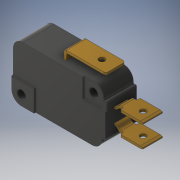
# Autodesk Inventor part: fc17-076
Saved by Autodesk Inventor 2017.1 (Build 211199000, 199)
## iProperties
Category: Electrical
Company: Autodesk Inc.
Created: 2016-12-17
Part Number: fc17-076
Material: Generic
Document SubType Name: Modeling
Designer: Autodesk Inc.
Density: 1 g/cm^3
Appearance: Default
Catalog Web Link: http://www.mouser.com/ds/2/187/honeywell-sensing-micro-switch-V7-basic-product-sh-740331.pdf
Vendor: Honeywell
Author: Autodesk Inc.
Keywords: FIRST Choice
Autodesk Inventor part; units mm, degrees
sketch "Sketch1" plane through (0, 0, 0) normal (0, 1, 0) x (-1, 0, 0)
  line L0 (0, 0) -> (0, -48.4764) construction
  line L1 (0, -48.4764) -> (-27.2974, -48.4764) construction
  line L2 (-27.2974, -48.4764) -> (-27.2974, 0) construction
  line L3 (-27.2974, 0) -> (0, 0) construction
  line L4 (-4.6059, -3.65) -> (-22.1318, -3.65)
  line L5 (-22.1318, -3.65) -> (-22.1318, -32.3372)
  line L6 (-22.1318, -32.3372) -> (-4.6059, -32.3372)
  line L7 (-4.6059, -32.3372) -> (-4.6059, -3.65)
  line L8 (-8.3878, -32.3372) -> (-18.7189, -32.3372)
  line L9 (-18.7189, -32.3372) -> (-18.7189, -33.368)
  line L10 (-18.7189, -33.368) -> (-8.3878, -33.368)
  line L11 (-8.3878, -33.368) -> (-8.3878, -32.3372)
  line L12 (-15.2137, -3.65) -> (-15.2137, -10.9371)
  line L13 (-15.2137, -10.9371) -> (-22.1318, -10.9371)
  line L14 (-10.7861, -32.3372) -> (-10.7861, -26.0648)
  line L15 (-10.7861, -26.0648) -> (-4.6059, -26.0648)
  dimension "d15" = 29.718
  constraints: 24 end point, 5 perpendicular, 5 point on line, 4 parallel, 2 horizontal, 1 vertical, 2 other
  measures "d15" vertical distance of L9.end L4.end
extrude "Extrusion1" add sketch "Sketch1" against normal blind 10.16 contours L7 L15 L14 L6 L5 L13 L12 L4 | L12 L13 L5 L4 | L7 L6 L14 L15
fillet "Fillet1" radius 3.175 4 edges at (4.6059, -5.08, -3.65) (22.1318, -5.08, -3.65) (22.1318, -5.08, -32.3372) (4.6059, -5.08, -32.3372)
extrude "Extrusion2" add sketch "Sketch1" against normal up to surface (10.16 mm away) contours L11 L10 L9 L6
fillet "Fillet2" radius 0.254 4 edges at (8.3878, -5.08, -32.3372) (8.3878, -5.08, -33.368) (18.7189, -5.08, -33.368) (18.7189, -5.08, -32.3372)
sketch "Sketch2" plane through (0, 0, 0) normal (0, 1, 0) x (1, 0, 0)
  arc A0 (7.7809, 32.3372) -> (4.6059, 29.1622) centre (7.7809, 29.1622) ccw projected
  arc A1 (18.9568, 3.65) -> (22.1318, 6.825) centre (18.9568, 6.825) ccw projected
  point P0 (0, 0)
hole "Hole1" at (7.7809, 0, -29.1622) at (18.9568, 0, -6.825) direction (0, -1, 0) diameter 2.794 end through all
sketch "Sketch3" plane through (0, 0, 0) normal (0, 1, 0) x (1, 0, 0)
  arc A0 (7.7809, 32.3372) -> (4.6059, 29.1622) centre (7.7809, 29.1622) ccw projected
  arc A1 (18.9568, 3.65) -> (22.1318, 6.825) centre (18.9568, 6.825) ccw projected
  circle A2 centre (18.9568, 6.825) radius 1.397 projected
  circle A3 centre (7.7809, 29.1622) radius 1.397 projected
  point P0 (0, 0)
sketch "Sketch4" plane through (0, 0, 0) normal (0, 1, 0) x (1, 0, 0)
  line L0 (7.7809, 3.65) -> (18.9568, 3.65) projected
  line L1 (15.242, 3.65) -> (15.242, 3.65)
  line L2 (15.242, 3.65) -> (18.9568, 3.65)
  line L3 (22.1318, 6.825) -> (22.1318, 29.1622) projected
  arc A0 (18.9568, 3.65) -> (22.1318, 6.825) centre (18.9568, 6.825) ccw projected
  line L4 (18.9568, 3.65) -> (15.242, 3.65)
  circle A1 centre (18.9568, 6.825) radius 1.397 projected
  line L5 (15.2137, 3.65) -> (15.2137, 10.9371) projected
  line L6 (15.2137, 10.9371) -> (22.1318, 10.9371) projected
  line L7 (15.2137, 3.65) -> (15.2137, 10.9371)
  line L8 (4.6059, 6.825) -> (4.6059, 29.1622) projected
  line L9 (15.2137, 10.9371) -> (22.1318, 10.9371)
  line L10 (22.1318, 10.9371) -> (22.1318, 6.825)
  line L11 (18.9568, 3.65) -> (15.2137, 3.65)
  point P0 (0, 0)
  constraints: 14 end point, 3 perpendicular, 2 point on circle, 1 collinear, 1 parallel, 1 point on line, 1 tangent, 1 vertical
extrude "Extrusion4" add sketch "Sketch4" along normal blind 0.508
fillet "Fillet3" radius 0.127 4 edges at (15.2137, 0, -7.2936) (15.2137, 0.508, -7.2936) (18.6728, 0, -10.9371) (18.6728, 0.508, -10.9371)
sketch "Sketch6" plane through (0, 0, 0) normal (0, 1, 0) x (1, 0, 0)
  line L0 (4.6059, 26.1612) -> (10.8013, 26.1612)
  line L1 (10.8013, 26.1612) -> (10.8013, 32.3448)
  line L2 (4.6059, 29.1622) -> (4.6059, 26.1612)
  line L3 (10.8013, 32.3448) -> (10.8013, 33.368)
  line L4 (18.4649, 33.368) -> (8.6418, 33.368) projected
  line L5 (10.8013, 33.368) -> (8.6418, 33.368)
  line L6 (4.6059, 29.1622) -> (4.6059, 6.825) projected
  arc A0 (7.7809, 32.3372) -> (4.6059, 29.1622) centre (7.7809, 29.1622) ccw projected
  line L7 (7.7809, 32.3372) -> (8.1338, 32.3372) projected
  line L8 (7.7809, 32.3372) -> (8.1338, 32.3372)
  arc A1 (8.1338, 32.3372) -> (8.3878, 32.5912) centre (8.1338, 32.5912) ccw projected
  line L9 (8.3878, 32.5912) -> (8.3878, 33.114)
  line L10 (8.3878, 33.114) -> (8.3878, 32.5912) projected
  arc A2 (8.1338, 32.3372) -> (8.3878, 32.5912) centre (8.1338, 32.5912) ccw
  arc A3 (8.6418, 33.368) -> (8.3878, 33.114) centre (8.6418, 33.114) ccw projected
  arc A4 (8.6418, 33.368) -> (8.3878, 33.114) centre (8.6418, 33.114) ccw
  point P0 (0, 0)
  constraints: 17 end point, 6 point on circle, 3 collinear, 2 centre point, 2 coincident, 2 concentric, 2 horizontal, 1 parallel, 1 perpendicular, 1 point on line, 1 vertical
extrude "Extrusion5" cut sketch "Sketch6" against normal blind 0.508
fillet "Fillet4" radius 0.127 14 edges at (5.5358, -0.508, -31.4073) (7.9573, -0.508, -32.3372) (8.3134, -0.508, -32.4116) (8.3878, -0.508, -32.8526) (8.4622, -0.508, -33.2936) (9.7215, -0.508, -33.368) (4.6059, -0.508, -27.6617) (10.8013, -0.254, -33.368) (10.8013, 0, -29.7646) (10.8013, -0.508, -29.7646) (10.8013, -0.254, -26.1612) (7.7036, -0.508, -26.1612) (7.7036, 0, -26.1612) (4.6059, -0.254, -26.1612)
ref_plane "Work Plane2" through (9.5334, -10.16, -6.825) normal (-1, 0, 0) x (0, 0, 1)
ref_plane "Work Plane1" through (13.3688, -10.16, -6.825) normal (-1, 0, 0) x (0, 0, 1)
ref_plane "Work Plane3" through (0, -5.08, 0) normal (0, 1, 0) x (1, 0, 0)
sketch "Sketch9" plane through (0, -5.08, 0) normal (0, 1, 0) x (1, 0, 0)
  line L0 (9.5334, -6.6736) -> (9.5334, 40.0416) projected
  circle A0 centre (7.7809, 29.1622) radius 1.397 projected
  line L1 (9.5334, 33.368) -> (9.5334, 42.8385)
  line L2 (10.2954, 33.368) -> (10.2954, 42.8385)
  line L3 (10.6743, 33.368) -> (8.6418, 33.368) projected
  line L4 (10.9283, 33.368) -> (10.6743, 33.368) projected
  line L5 (18.4649, 33.368) -> (10.9283, 33.368) projected
  line L6 (9.7239, 43.6402) -> (10.1049, 43.6402)
  line L7 (9.5334, 42.8385) -> (9.7239, 43.6402)
  line L8 (10.2954, 42.8385) -> (10.1049, 43.6402)
  line L9 (10.2954, 35.0309) -> (11.3926, 34.062)
  line L10 (11.3926, 34.062) -> (11.3926, 33.368)
  line L11 (9.5334, 35.0309) -> (10.844, 33.8736)
  line L12 (10.844, 33.368) -> (10.844, 33.8736)
  point P0 (0, 0)
  dimension "d43" = 14.478
  dimension "d44" = 0.762
  dimension "d47" = 0.381
  dimension "d48" = 0.1905
  constraints: 18 end point, 6 point on line, 3 parallel, 1 collinear, 1 horizontal, 1 perpendicular, 1 vertical
  measures "d43" vertical distance of L6.start A0.centre
  measures "d44" distance between parallel lines of L2 L1
  measures "d47" distance of L6.start L6.end
  measures "d48" horizontal distance of L6.end L2.end
extrude "Extrusion6" add sketch "Sketch9" along normal mid plane 6.35 contours L0 L1 L7 L6 L8 L2 L11 | L2 L9 L10 L5 L4 L12 L11
fillet "Fillet5" radius 1.27 4 edges at (9.5334, -5.08, -35.0309) (10.844, -5.08, -33.8736) (10.2954, -5.08, -35.0309) (11.3926, -5.08, -34.062)
sketch "Sketch10" plane through (9.5334, -8.255, -42.8385) normal (-1, 0, 0) x (0, 0, 1)
  line L0 (6.4322, 0) -> (9.4705, 0)
  line L1 (9.4705, 0) -> (9.4705, 1.074)
  line L2 (9.4705, 1.074) -> (6.4322, 1.074)
  line L3 (6.4322, 1.074) -> (6.4322, 0)
  line L4 (0, 6.35) -> (7.2348, 6.35) projected
  line L5 (6.4322, 6.35) -> (9.4705, 6.35)
  line L6 (9.4705, 6.35) -> (9.4705, 5.276)
  line L7 (9.4705, 5.276) -> (6.4322, 5.276)
  line L8 (6.4322, 5.276) -> (6.4322, 6.35)
  line L9 (9.4705, 7.62) -> (9.4705, -1.905) projected
  line L10 (7.2348, 0) -> (0, 0) projected
  point P0 (42.8385, 8.255)
  constraints: 16 end point, 4 collinear, 4 parallel, 2 horizontal, 2 perpendicular, 2 point on line
extrude "Extrusion7" cut sketch "Sketch10" against normal blind 3.175
fillet "Fillet6" radius 0.254 4 edges at (9.9144, -1.905, -36.4063) (9.9144, -2.979, -36.4063) (9.9144, -7.181, -36.4063) (9.9144, -8.255, -36.4063)
sketch "Sketch11" plane through (9.5334, -8.255, -42.8385) normal (-1, 0, 0) x (0, 0, 1)
  line L0 (-0.8017, 0) -> (-0.8017, 6.35) projected
  point P0 (42.8385, 8.255)
  point P1 (2.248, 3.175)
  point P2 (-0.8017, 3.175)
  constraints: 1 horizontal alignment, 1 midpoint
hole "Hole2" at (9.5334, -5.08, -40.5905) direction (1, 0, 0) diameter 1.905 end through all
mirror "Mirror1" about plane through (13.3688, -10.16, -6.825) normal (-1, 0, 0) of "Extrusion6", "Hole2", "Extrusion7", "Fillet6", "Fillet5"
ref_plane "Work Plane5" through (2.4468, -35.9659, -6.825) normal (1, 0, 0) x (0, 1, 0)
ref_plane "Work Plane4" through (18.9568, -35.9659, -6.825) normal (1, 0, 0) x (0, 1, 0)
sketch "Sketch12" plane through (2.4468, -35.9659, -6.825) normal (1, 0, 0) x (0, 1, 0)
  line L0 (35.5849, -19.2092) -> (35.9659, -19.2092) projected
  arc A0 (35.5849, -19.2092) -> (35.3309, -19.4632) centre (35.5849, -19.4632) ccw projected
  line L1 (35.3309, -22.3372) -> (35.3309, -19.4632) projected
  line L2 (25.8059, -22.3372) -> (35.3309, -22.3372) projected
  line L3 (25.8059, 0) -> (25.8059, -22.3372) projected
  line L4 (35.9659, 0) -> (25.8059, 0) projected
  line L5 (35.9659, -19.2092) -> (35.9659, 0) projected
  line L6 (27.7109, -12.0957) -> (34.0609, -12.0957)
  line L7 (34.0609, -12.0957) -> (34.0609, -24.8546)
  line L8 (34.0609, -24.8546) -> (27.7109, -24.8546)
  line L9 (27.7109, -24.8546) -> (27.7109, -12.0957)
  line L10 (35.3309, -26.543) -> (25.8059, -26.543) projected
  point P0 (35.9659, 6.825)
  dimension "d64" = 10.16
  dimension "d65" = 6.35
  dimension "d66" = 1.905
  constraints: 8 end point, 2 parallel, 1 horizontal, 1 perpendicular
  measures "d64" distance of L4.start L3.start
  measures "d65" distance of L6.start L6.end
  measures "d66" distance between parallel lines of L9 L3
extrude "Extrusion8" add sketch "Sketch12" against normal blind 0.762 contours L7 L8 L9 L2 | L2 L9 L6 L7
sketch "Sketch13" plane through (2.4468, -8.255, -18.9207) normal (0, 0, 1) x (1, 0, 0)
  line L0 (-0.762, 0) -> (-0.762, 6.35) projected
  line L1 (-0.762, 0) -> (2.1591, 0)
  line L2 (2.1591, 0) -> (2.1591, 6.3398)
  line L3 (2.1591, 6.3398) -> (-0.762, 6.3398)
  line L4 (-0.762, 6.3398) -> (-0.762, 0)
  line L5 (2.1591, 8.255) -> (2.1591, -1.905) projected
  point P0 (-2.4468, 8.255)
  constraints: 8 end point, 2 parallel, 1 collinear, 1 horizontal, 1 perpendicular
extrude "Extrusion9" add sketch "Sketch13" along normal blind 0.762
fillet "Fillet7" radius 0.762 1 edges at (1.6848, -5.0851, -18.1587)
fillet "Fillet8" radius 0.762 1 edges at (2.4468, -5.0851, -18.9207)
sketch "Sketch14" plane through (1.6848, -35.9659, -6.825) normal (-1, 0, 0) x (0, 0, 1)
  point P0 (6.825, 35.9659)
  point P1 (-20.4324, 30.8859)
hole "Hole3" at (1.6848, -5.08, -27.2574) direction (1, 0, 0) diameter 1.905 end up to surface
fillet "Fillet9" radius 0.762 2 edges at (2.0658, -1.905, -31.6796) (2.0658, -8.255, -31.6796)
body "Solid1"
